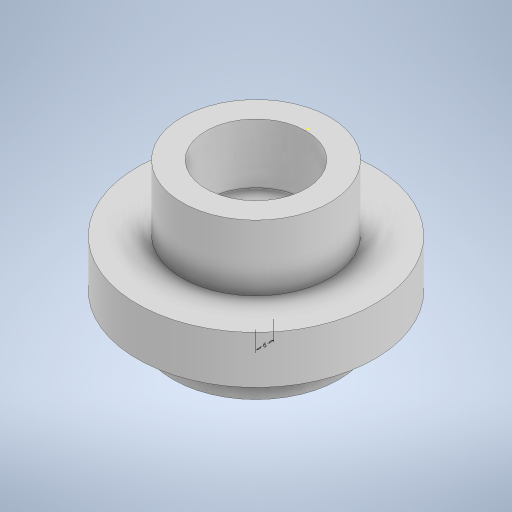
# Autodesk Inventor part: Задание номер 3
Saved by Autodesk Inventor 2023.2 (Build 272271030, 271C)
## iProperties
Created: 2023-09-07
Part Number: Задание номер 3
Material: Типовые
Document SubType Name: Modeling
Designer: User
Density: 1 g/cm^3
Appearance: По умолчанию
Author: User
Autodesk Inventor part; units mm, degrees
ref_plane "YZ Plane" through (0, 0, 0) normal (1, 0, 0) x (0, 1, 0)
ref_plane "XZ Plane" through (0, 0, 0) normal (0, 1, 0) x (-1, 0, 0)
ref_plane "XY Plane" through (0, 0, 0) normal (0, 0, 1) x (1, 0, 0)
sketch "Эскиз1" plane through (0, 0, 0) normal (1, 0, 0) x (0, 1, 0)
  line L0 (-20.211, 11.7625) -> (-20.211, 0.7625)
  line L1 (-20.211, 0.7625) -> (-0.211, 0.7625)
  line L2 (-0.211, 0.7625) -> (-0.211, -7.2375)
  line L3 (-0.211, -7.2375) -> (-22.211, -7.2375)
  line L4 (-22.211, -7.2375) -> (-22.211, -22.2375)
  line L5 (-20.211, 11.7625) -> (-50.211, 11.7625)
  line L6 (-50.211, 11.7625) -> (-50.211, 5.7625)
  line L7 (-50.211, 5.7625) -> (-42.211, 5.7625)
  line L8 (-42.211, 5.7625) -> (-42.211, -2.2375)
  line L9 (-42.211, -2.2375) -> (-50.211, -2.2375)
  line L10 (-50.211, -2.2375) -> (-50.211, -10.2375)
  line L11 (-50.211, -10.2375) -> (-38.211, -10.2375)
  line L12 (-38.211, -10.2375) -> (-38.211, -22.2375)
  line L13 (-38.211, -22.2375) -> (-22.211, -22.2375)
  point P0 (0, 0)
  dimension "d0" = 15
  dimension "d1" = 22
  dimension "d2" = 20
  dimension "d3" = 11
  dimension "d4" = 12
  dimension "d5" = 12
  dimension "d6" = 8
  dimension "d7" = 6
  dimension "d8" = 50
  dimension "d9" = 50
  dimension "d10" = 34
  dimension "d11" = 8
  constraints: 28 end point, 12 perpendicular, 1 horizontal, 1 vertical
  measures "d0" distance of L3.end L4.end
  measures "d1" distance of L2.end L3.end
  measures "d2" distance of L0.end L1.end
  measures "d3" distance of L0.start L0.end
  measures "d4" distance of L10.end L11.end
  measures "d5" distance of L11.end L12.end
  measures "d6" distance of L7.end L8.end
  measures "d7" distance of L5.end L6.end
  measures "d8" distance from line of L10 L2.end
  measures "d9" horizontal distance of L1.end L5.end
  measures "d10" vertical distance of L12.end L5.end
  measures "d11" distance of L6.end L7.end
sketch "Эскиз2" plane through (0, 0, 0) normal (1, 0, 0) x (0, 1, 0)
  line L0 (-49.3354, 11.5668) -> (-49.3354, 17.5668)
  line L1 (-49.3354, 17.5668) -> (-14.2528, 17.5668)
  point P0 (0, 0)
  dimension "d12" = 6
  constraints: 4 end point, 1 perpendicular, 1 vertical
  measures "d12" distance of L0.start L0.end
revolve "Вращение1" add sketch "Эскиз1" angle 360 about axis through (0, -49.3354, 17.5668) along (0, 1, 0)
